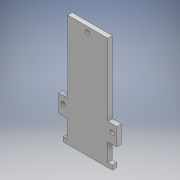
# Autodesk Inventor part: k2_t_l4
Saved by Autodesk Inventor 2017 (Build 210142000, 142)
## iProperties
Created: 2017-02-10
Part Number: k2_t_l4
Material: Generic
Document SubType Name: Modeling
Designer: herman
Density: 1 g/cm^3
Appearance: Default
d2: 3,000 mm
d3: 0,00 deg
d8: 3,000 mm
d9: 3,000 mm
d11: 33,000 mm
d12: 12,000 mm
d13: 60,415 mm
d14: 12,000 mm
Author: herman
Autodesk Inventor part; units mm, degrees
ref_plane "YZ Plane" through (0, 0, 0) normal (1, 0, 0) x (0, 1, 0)
ref_plane "XZ Plane" through (0, 0, 0) normal (0, 1, 0) x (-1, 0, 0)
ref_plane "XY Plane" through (0, 0, 0) normal (0, 0, 1) x (1, 0, 0)
sketch "Sketch1" plane through (0, 0, 0) normal (0, 1, 0) x (-1, 0, 0)
  line L0 (16.2379, 4.3509) -> (-10.7621, 4.3509)
  line L1 (-13.7621, -68.0643) -> (-13.7621, -71.0643)
  line L2 (-13.7621, -71.0643) -> (19.2379, -71.0643)
  line L3 (19.2379, -71.0643) -> (19.2379, -68.0643)
  line L4 (22.2379, -56.0643) -> (16.2379, -56.0643)
  line L5 (16.2379, -56.0643) -> (16.2379, -68.0643)
  line L6 (16.2379, -68.0643) -> (19.2379, -68.0643)
  line L7 (-13.7621, -68.0643) -> (-10.7621, -68.0643)
  line L8 (-10.7621, -68.0643) -> (-10.7621, -56.0643)
  line L9 (-10.7621, -56.0643) -> (-16.7621, -56.0643)
  line L10 (22.2379, -56.0643) -> (22.2379, -44.0643)
  line L11 (22.2379, -44.0643) -> (16.2379, -44.0643)
  line L12 (16.2379, -44.0643) -> (16.2379, 4.3509)
  line L13 (-16.7621, -56.0643) -> (-16.7621, -44.0643)
  line L14 (-16.7621, -44.0643) -> (-10.7621, -44.0643)
  line L15 (-10.7621, -44.0643) -> (-10.7621, 4.3509)
  dimension "d8" = 3
  dimension "d9" = 3
  dimension "d11" = 33
  dimension "d12" = 12
  dimension "d13" = 60.4152
  dimension "d14" = 12
  dimension "d24" = 6
  dimension "d25" = 6
  constraints: 32 end point, 10 perpendicular, 5 equal length, 2 horizontal, 2 point on line, 2 vertical, 1 parallel
  measures "d8" distance of L5.end L3.end
  measures "d9" distance of L2.end L3.end
  measures "d11" distance of L1.end L2.end
  measures "d12" distance of L4.start L10.end
  measures "d13" distance of L0.start L4.end
  measures "d14" distance of L4.end L5.end
  measures "d24" distance of L8.end L9.end
  measures "d25" distance of L4.start L4.end
extrude "Extrusion1" add sketch "Sketch1" along normal blind 3
sketch "Sketch5" plane through (0, 3, 0) normal (0, 1, 0) x (1, 0, 0)
  circle A0 centre (13.7621, 49.0643) radius 1.496
  circle A1 centre (-19.2379, 49.0643) radius 1.5213
  circle A2 centre (-2.7379, -0.9357) radius 1.5
  line L0 (10.7621, 44.0643) -> (16.7621, 44.0643) projected
  line L1 (16.7621, 44.0643) -> (16.7621, 56.0643) projected
  line L2 (-22.2379, 44.0643) -> (-16.2379, 44.0643) projected
  line L3 (-22.2379, 56.0643) -> (-22.2379, 44.0643) projected
  line L4 (10.7621, -4.3509) -> (10.7621, 44.0643) projected
  line L5 (-16.2379, -4.3509) -> (10.7621, -4.3509) projected
  line L6 (13.7621, 71.0643) -> (-19.2379, 71.0643) projected
  point P0 (0, 0)
  dimension "d36" = 5
  dimension "d37" = 3
  dimension "d38" = 5
  dimension "d39" = 3
  dimension "d41" = 13.5
  dimension "d42" = 3
  dimension "d46" = 72
  constraints: 3 centre point
  measures "d36" distance from line of L0 A0.centre
  measures "d37" distance from line of L1 A0.centre
  measures "d38" distance from line of L2 A1.centre
  measures "d39" distance from line of L3 A1.centre
  measures "d41" distance from line of L4 A2.centre
  measures "d42" diameter of A2
  measures "d46" distance from line of A2.centre L6
extrude "Extrusion2" cut sketch "Sketch5" against normal through all
body "Solid1"
